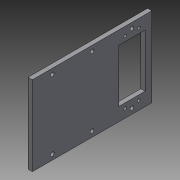
# Autodesk Inventor part: ServoPlate1
Saved by Autodesk Inventor 2014 SP1 (Build 180222100, 222)
## iProperties
Created: 2014-11-10
Part Number: ServoPlate1
Material: Generic
Document SubType Name: Modeling
Designer: rawrdong
Density: 1 g/cm^3
Appearance: Default
Author: rawrdong
Autodesk Inventor part; units mm, degrees
ref_plane "YZ Plane" through (0, 0, 0) normal (1, 0, 0) x (0, 1, 0)
ref_plane "XZ Plane" through (0, 0, 0) normal (0, 1, 0) x (-1, 0, 0)
ref_plane "XY Plane" through (0, 0, 0) normal (0, 0, 1) x (1, 0, 0)
sketch "Sketch1" plane through (0, 0, 0) normal (1, 0, 0) x (0, 1, 0)
  line L0 (0, 0) -> (90, 0)
  line L1 (90, 0) -> (90, -60)
  line L2 (90, -60) -> (0, -60)
  line L3 (0, -60) -> (0, 0)
  circle A0 centre (15, -4) radius 1.425
  circle A1 centre (45, -4) radius 1.425
  circle A2 centre (75, -4) radius 1.425
  line L4 (0, -4) -> (90, -4) construction
  line L5 (45, -60) -> (45, 0) construction
  line L6 (0, -30) -> (90, -30) construction
  circle A3 centre (15, -56) radius 1.425
  circle A4 centre (45, -56) radius 1.425
  circle A5 centre (75, -56) radius 1.425
  dimension "d0" = 2.85
  dimension "d1" = 90
  dimension "d2" = 30
  dimension "d3" = 4
  dimension "d4" = 60
  constraints: 14 end point, 6 centre point, 5 midpoint, 5 point on line, 4 symmetric about line, 2 equal radius, 2 parallel, 2 perpendicular, 1 horizontal, 1 vertical, 3 other
  measures "d0" diameter of A1
  measures "d1" distance of L0.start L0.end
  measures "d2" distance of A1.centre A0.centre
  measures "d3" distance between parallel lines of L0 L4
  measures "d4" distance of L0.end L1.end
extrude "Extrusion1" add sketch "Sketch1" along normal blind 3.2
sketch "Sketch2" plane through (3.2, 0, 0) normal (1, 0, 0) x (0, 0, -1)
  circle A0 centre (56, 75) radius 1.425 projected
  circle A1 centre (4, 75) radius 1.425 projected
  line L0 (60, 90) -> (0, 90) projected
  line L1 (30, 90) -> (30, -95.4624)
  line L2 (10.06, 84.91) -> (49.94, 84.91)
  line L3 (49.94, 84.91) -> (49.94, 65.09)
  line L4 (49.94, 65.09) -> (10.06, 65.09)
  line L5 (10.06, 65.09) -> (10.06, 84.91)
  line L6 (4, 75) -> (56, 75) construction
  circle A2 centre (6.37, 80.085) radius 1.05
  circle A3 centre (6.37, 69.915) radius 1.05
  circle A4 centre (53.63, 80.085) radius 1.05
  circle A5 centre (53.63, 69.915) radius 1.05
  point P0 (49.94, 75)
  dimension "d7" = 39.88
  dimension "d8" = 19.82
  dimension "d9" = 10.17
  dimension "d10" = 47.26
  dimension "d11" = 2.1
  constraints: 12 end point, 4 centre point, 3 equal radius, 3 perpendicular, 3 symmetric about line, 2 midpoint, 2 parallel, 1 horizontal, 1 point on line, 1 other
  measures "d7" distance of L2.start L2.end
  measures "d8" distance of L4.end L2.start
  measures "d9" distance of A2.centre A3.centre
  measures "d10" distance of A2.centre A4.centre
  measures "d11" diameter of A2
extrude "Extrusion2" cut sketch "Sketch2" against normal through all contours L2 L3 L4 L1 | L1 L4 L5 L2 | A2 | A3 | A4 | A5
body "Solid1"
